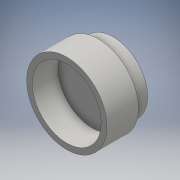
# Autodesk Inventor part: magnet_holder
Saved by Autodesk Inventor 2016 (Build 200138000, 138)
## iProperties
Created: 2017-06-18
Part Number: magnet_holder
Material: Ogólny
Document SubType Name: Modeling
Designer: Karol
Density: 1 g/cm^3
Appearance: Domyślna
Author: Karol
Autodesk Inventor part; units mm, degrees
ref_plane "YZ Plane" through (0, 0, 0) normal (1, 0, 0) x (0, 1, 0)
ref_plane "XZ Plane" through (0, 0, 0) normal (0, 1, 0) x (-1, 0, 0)
ref_plane "XY Plane" through (0, 0, 0) normal (0, 0, 1) x (1, 0, 0)
sketch "Sketch1" plane through (0, 0, 0) normal (0, 1, 0) x (-1, 0, 0)
  line L0 (0, -2.3094) -> (-2, -1.1547)
  line L1 (-2, -1.1547) -> (-2, 1.1547)
  line L2 (-2, 1.1547) -> (0, 2.3094)
  line L3 (0, 2.3094) -> (2, 1.1547)
  line L4 (2, 1.1547) -> (2, -1.1547)
  line L5 (2, -1.1547) -> (0, -2.3094)
  circle A0 centre (0, 0) radius 3
  circle A1 centre (0, 0) radius 3.5
  dimension "d0" = 4
  dimension "d1" = 6
  dimension "d4" = 7
  constraints: 12 end point, 3 coincident, 2 centre point, 13 other
  measures "d0" distance between parallel lines of L5 L2
  measures "d1" diameter of A0
  measures "d4" diameter of A1
extrude "Extrusion1" add sketch "Sketch1" along normal blind 1.3 contours A0
extrude "Extrusion2" add sketch "Sketch1" against normal blind 0.5 contours L0 L1 L2 L3 L4 L5 | A0 | A1
ref_plane "Work Plane1" through (0, -0.25, 0) normal (0, -1, 0) x (1, 0, 0)
sketch "Sketch2" plane through (0, -0.25, 0) normal (0, -1, 0) x (1, 0, 0)
  line L0 (0, -2.3094) -> (-2, -1.1547) projected
  line L1 (0, -2.3094) -> (2, -1.1547) projected
  line L2 (2, 1.1547) -> (2, -1.1547) projected
  line L3 (2, 1.1547) -> (0, 2.3094) projected
  line L4 (-2, 1.1547) -> (0, 2.3094) projected
  line L5 (-2, 1.1547) -> (-2, -1.1547) projected
  line L6 (-2, -1.1547) -> (0, -2.3094) projected
  circle A0 centre (0, 0) radius 3.5 projected
  circle A1 centre (0, 0) radius 3 projected
extrude "Extrusion3" add sketch "Sketch2" along normal blind 2.5 contours A0
body "Solid1"
